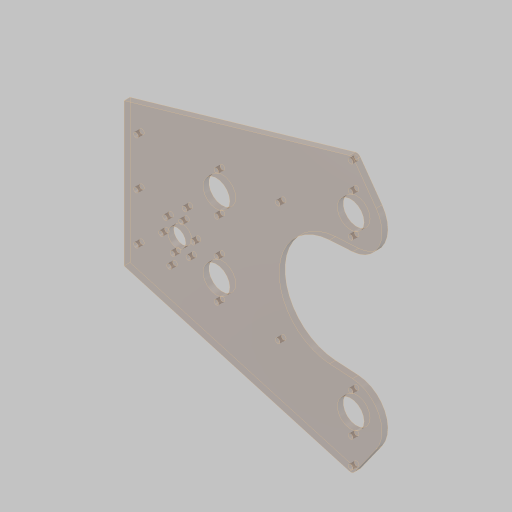
# Autodesk Inventor part: GP6-001
Saved by Autodesk Inventor 2023.5 (Build 275446000, 446)
## iProperties
Created: 2025-02-23
Part Number: GP6-001
Material: Polycarbonate, Smoke
Document SubType Name: Modeling
Designer: slick
Density: 1.2 g/cm^3
Appearance: Polycarbonate - Smoked
Author: slick
Autodesk Inventor part; units mm, degrees
ref_plane "YZ Plane" through (0, 0, 0) normal (1, 0, 0) x (0, 1, 0)
ref_plane "XZ Plane" through (0, 0, 0) normal (0, 1, 0) x (-1, 0, 0)
ref_plane "XY Plane" through (0, 0, 0) normal (0, 0, 1) x (1, 0, 0)
sketch "Sketch1" plane through (0, 0, 0) normal (0, 0, 1) x (1, 0, 0)
  circle A0 centre (0, 91.8009) radius 38.1 construction
  circle A1 centre (0, -91.8009) radius 38.1 construction
  line L0 (0, 91.8009) -> (0, -91.8009) construction
  circle A2 centre (-25.4, 0) radius 57.15 construction
  circle A3 centre (0, 91.8009) radius 14.2875
  circle A4 centre (0, -91.8009) radius 14.2875
  circle A5 centre (0, -91.8009) radius 33.3375 construction
  circle A6 centre (0, 91.8009) radius 33.3375 construction
  circle A7 centre (-142.9967, -39.6875) radius 14.3256 construction
  circle A8 centre (0, -91.8009) radius 23.876 construction
  line L1 (-142.9967, -39.6875) -> (0, -91.8009) construction
  circle A9 centre (-142.9967, 39.6875) radius 14.3256 construction
  circle A10 centre (0, 91.8009) radius 23.876 construction
  line L2 (0, 91.8009) -> (-142.9967, 39.6875) construction
  circle A11 centre (-142.9967, 39.6875) radius 39.6875 construction
  circle A12 centre (-142.9967, -39.6875) radius 39.6875 construction
  line L3 (-142.9967, 39.6875) -> (-142.9967, -39.6875) construction
  line L4 (-138.9458, 25.9466) -> (6.7516, 68.8994) construction
  line L5 (-9.5669, 113.6764) -> (-148.7368, 52.8128) construction
  line L6 (-138.9458, -25.9466) -> (6.7516, -68.8994) construction
  circle A13 centre (-142.9967, 39.6875) radius 14.2875
  circle A14 centre (-142.9967, -39.6875) radius 14.2875
  circle A15 centre (-185.1646, -22.225) radius 5.9531 construction
  circle A16 centre (-185.1646, -22.225) radius 9.525
  circle A17 centre (-185.1646, -22.225) radius 17.4625 construction
  circle A18 centre (-185.1646, -22.225) radius 17.4625 construction
  circle A19 centre (-185.1646, -22.225) radius 17.4625 construction
  circle A20 centre (-185.1646, -22.225) radius 17.4625 construction
  circle A21 centre (-185.1646, -22.225) radius 17.4625 construction
  circle A22 centre (-19.05, 0) radius 57.15 construction
  circle A23 centre (-185.1646, -22.225) radius 19.05 construction
  line L7 (-241.3, 76.2) -> (-215.9, 76.2) construction
  line L8 (-215.9, 76.2) -> (-215.9, -76.2) construction
  line L9 (-215.9, -76.2) -> (-241.3, -76.2) construction
  line L10 (-241.3, -76.2) -> (-241.3, 76.2)
  line L11 (-142.9967, -39.6875) -> (-185.1646, -22.225) construction
  line L12 (-77.6563, 63.5) -> (-77.6563, -63.5) construction
  line L13 (-22.4906, -57.0463) -> (2.007, -58.5239)
  arc A24 (2.007, 58.5239) -> (27.142, 111.1581) centre (0, 91.8009) ccw
  arc A25 (-22.4906, 57.0463) -> (-22.4906, -57.0463) centre (-19.05, 0) ccw
  line L14 (2.007, 58.5239) -> (-22.4906, 57.0463)
  arc A26 (27.142, -111.1581) -> (2.007, -58.5239) centre (0, -91.8009) ccw
  arc A27 (3.8774, 143.7787) -> (-1.3229, 145.5885) centre (0, 141.0134) ccw
  circle A28 centre (0, 91.8009) radius 44.45 construction
  line L15 (3.8774, 143.7787) -> (27.142, 111.1581)
  line L16 (-1.3229, 145.5885) -> (-241.3, 76.2)
  arc A29 (-1.3229, -145.5885) -> (3.8774, -143.7787) centre (0, -141.0134) ccw
  line L17 (-241.3, -76.2) -> (-1.3229, -145.5885)
  line L18 (27.142, -111.1581) -> (3.8774, -143.7787)
  circle A30 centre (0, -91.8009) radius 44.45 construction
  line L19 (0, 112.8194) -> (0, 70.7824) construction
  line L20 (-142.9967, 60.706) -> (-142.9967, 18.669) construction
  line L21 (-142.9967, -18.669) -> (-142.9967, -60.706) construction
  line L22 (0, -70.7824) -> (0, -112.8194) construction
  line L23 (-228.6, 50.8) -> (-228.6, -50.8) construction
  line L24 (-176.9471, 8.4431) -> (-193.3821, -52.8931) construction
  circle A31 centre (-176.9471, 8.4431) radius 4.7625 construction
  line L25 (-148.7368, -52.8128) -> (-9.5669, -113.6764) construction
  line L26 (-185.1646, -22.225) -> (-180.6449, -5.3575) construction
  circle A32 centre (-185.1646, -22.225) radius 17.4625 construction
  point P0 (0, 0)
  point P1 (0, 0)
  point P2 (-168.2971, -17.7054)
  point P3 (-197.5124, -9.8771)
  point P4 (-202.032, -26.7446)
  point P5 (-189.6842, -39.0925)
  point P6 (-215.9, 0)
  point P7 (-228.6, 0)
  point P8 (-228.6, 0)
  point P9 (-228.6, 76.2)
  point P10 (-172.8167, -34.5729)
  dimension "d15" = 34.925
  dimension "d0" = 76.2
  dimension "d1" = 76.2
  dimension "d2" = 114.3
  dimension "d4" = 183.6018
  dimension "d5" = 28.575
  dimension "d6" = 19.05
  dimension "d7" = 28.6512
  dimension "d8" = 47.752
  dimension "d9" = 79.375
  dimension "d10" = 142.9967
  dimension "d11" = 152.1968
  dimension "d12" = 28.575
  dimension "d13" = 11.9062
  dimension "d14" = 19.05
  dimension "d18" = 360
  dimension "d20" = 6.35
  dimension "d21" = 38.1
  dimension "d22" = 25.4
  dimension "d23" = 152.4
  dimension "d24" = 241.3
  dimension "d26" = 127
  dimension "d29" = 9.525
  dimension "d30" = 6.35
  dimension "d32" = 42.037
  dimension "d33" = 42.037
  dimension "d34" = 42.037
  dimension "d35" = 42.037
  dimension "d36" = 25.4
  dimension "d44" = 101.6
  dimension "d45" = 63.5
  dimension "d47" = 9.525
  dimension "d48" = 15
  dimension "d49" = 53.975
  constraints: 54 end point, 27 centre point, 24 point on circle, 24 tangent, 20 coincident, 9 equal radius, 9 midpoint, 8 vertical, 3 horizontal alignment, 3 point on line, 3 vertical alignment, 2 parallel, 1 equal length, 1 horizontal, 1 perpendicular, 37 other
  measures "d0" diameter of A0
  measures "d1" diameter of A1
  measures "d2" diameter of A2
  measures "d4" distance of L0.start L0.end
  measures "d5" diameter of A3
  measures "d6" radial gap between concentric circles of A4 A5
  measures "d7" diameter of A7
  measures "d8" diameter of A8
  measures "d9" diameter of A11
  measures "d10" distance from line of L0.start L3
  measures "d11" distance of L2.end L2.start
  measures "d12" diameter of A13
  measures "d13" diameter of A15
  measures "d14" diameter of A16
  measures "d20" distance of A2.centre A22.centre
  measures "d21" diameter of A23
  measures "d22" distance of L8.end L9.end
  measures "d23" distance of L9.end L7.start
  measures "d24" distance from line of A3.centre L10
  measures "d26" distance of L12.start L12.end
  measures "d29" diameter of A27
  measures "d30" radial gap between concentric circles of A0 A28
  measures "d32" distance of L19.start L19.end
  measures "d33" distance of L20.start L20.end
  measures "d34" distance of L21.start L21.end
  measures "d35" distance of L22.start L22.end
  measures "d36" distance of point (0, 0) A2.centre
  measures "d44" distance of L23.start L23.end
  measures "d45" distance of L24.start L24.end
  measures "d47" diameter of A31
  measures "d48" angle of L8 L24
  measures "d49" distance from line of L11.end L9
extrude "Extrusion1" add sketch "Sketch1" along normal blind 6.35
hole "Hole1" at (-168.2971, -17.7054, 0) at (-180.6449, -5.3575, 0) at (-197.5124, -9.8771, 0) at (-202.032, -26.7446, 0) at (-189.6842, -39.0925, 0) at (-77.6563, 63.5, 0) at (-77.6563, -63.5, 0) at (0, 112.8194, 0) at (0, 70.7824, 0) at (-142.9967, 60.706, 0) at (-142.9967, 18.669, 0) at (-142.9967, -18.669, 0) at (-142.9967, -60.706, 0) at (0, -70.7824, 0) at (0, -112.8194, 0) at (-228.6, 50.8, 0) at (-228.6, 0, 0) at (-228.6, -50.8, 0) at (-176.9471, 8.4431, 0) at (-193.3821, -52.8931, 0) at (0, 141.0134, 0) at (0, -141.0134, 0) at (-172.8167, -34.5729, 0) direction (0, 0, 1) diameter 5.1054 end through all clearance for "Flat Head Machine Screw (82)" size "#10" standard "Ansi Unified Screw Threads"
body "Solid1"
